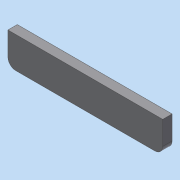
# Autodesk Inventor part: 0 零件
Saved by Autodesk Inventor 2020 (Build 240168000, 168)
## iProperties
Created: 2020-11-03
Part Number: 0 零件
Material: 一般
Document SubType Name: Modeling
Designer: p2013
Density: 1 g/cm^3
Appearance: 預設
Author: p2013
Autodesk Inventor part; units mm, degrees
ref_plane "YZ Plane" through (0, 0, 0) normal (1, 0, 0) x (0, 1, 0)
ref_plane "XZ Plane" through (0, 0, 0) normal (0, 1, 0) x (-1, 0, 0)
ref_plane "XY Plane" through (0, 0, 0) normal (0, 0, 1) x (1, 0, 0)
sketch "草圖1" plane through (0, 0, 0) normal (0, 0, 1) x (1, 0, 0)
  line L0 (0, 0) -> (-24.9363, 0) construction
  line L1 (0, 0) -> (0, 24.1407) construction
  line L2 (-22.25, -5) -> (22.25, -5)
  line L3 (24.75, -2.5) -> (24.75, 5)
  line L4 (24.75, 5) -> (-24.75, 5)
  line L5 (-24.75, 5) -> (-24.75, -2.5)
  line L6 (-24.75, -5) -> (24.75, 5) construction
  line L7 (24.75, -5) -> (-24.75, 5) construction
  arc A0 (22.25, -5) -> (24.75, -2.5) centre (22.25, -2.5) ccw
  arc A1 (-24.75, -2.5) -> (-22.25, -5) centre (-22.25, -2.5) ccw
  dimension "d0" = 49.5
  dimension "d1" = 10
  dimension "d4" = 2.5
  constraints: 16 end point, 4 point on circle, 4 point on line, 4 tangent, 2 centre point, 2 horizontal, 2 midpoint, 2 parallel, 1 equal radius, 1 perpendicular, 1 vertical
  measures "d0" distance between parallel lines of L3 L5
  measures "d1" distance between parallel lines of L2 L4
  measures "d4" radius of A0
extrude "擠出1" add sketch "草圖1" along normal mid plane 3
